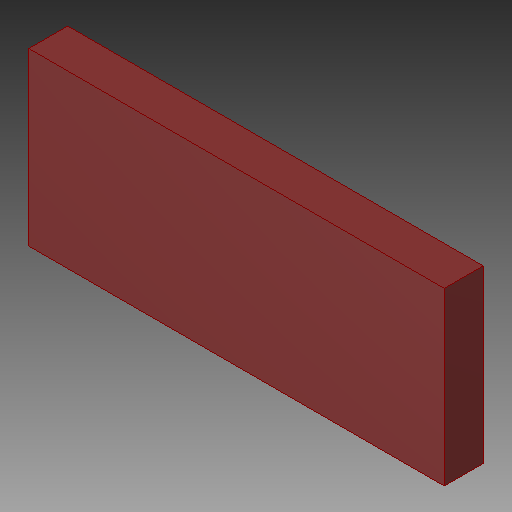
# Autodesk Inventor part: IC1_78XXS
Saved by Autodesk Inventor 2017 (Build 210142000, 142)
## iProperties
Created: 2019-06-13
Part Number: IC1_78XXS
Material: Generic
Document SubType Name: Modeling
Designer: Marc
Density: 1 g/cm^3
Appearance: 78XXS, IC1_78XXS
Author: Marc
Autodesk Inventor part; units mm, degrees
ref_plane "YZ Plane" through (0, 0, 0) normal (1, 0, 0) x (0, 1, 0)
ref_plane "XZ Plane" through (0, 0, 0) normal (0, 1, 0) x (-1, 0, 0)
ref_plane "XY Plane" through (0, 0, 0) normal (0, 0, 1) x (1, 0, 0)
sketch "78XXS, IC1_78XXS_22" plane through (0, 0, 0) normal (0, 0, 1) x (1, 0, 0)
  line L0 (-5.334, 0) -> (5.334, 0)
  line L1 (5.334, 0) -> (5.334, -4.3942)
  line L2 (5.334, -4.3942) -> (-5.334, -4.3942)
  line L3 (-5.334, -4.3942) -> (-5.334, 0)
  constraints: 8 end point
extrude "Extrusion1" add sketch "78XXS, IC1_78XXS_22" along normal blind 1
body "Solid1"
